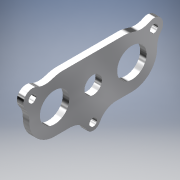
# Autodesk Inventor part: Gearbox Plate 1
Saved by Autodesk Inventor 2019.4 (Build 234330000, 330)
## iProperties
Created: 2019-12-11
Part Number: Gearbox Plate 1
Material: Aluminum 6061
Document SubType Name: Modeling
Designer: admin
Density: 2.7 g/cm^3
Appearance: Aluminum - Flat
Author: admin
Autodesk Inventor part; units mm, degrees
ref_plane "YZ Plane" through (0, 0, 0) normal (1, 0, 0) x (0, 1, 0)
ref_plane "XZ Plane" through (0, 0, 0) normal (0, 1, 0) x (-1, 0, 0)
ref_plane "XY Plane" through (0, 0, 0) normal (0, 0, 1) x (1, 0, 0)
sketch "Sketch6" plane through (0, 0, 0) normal (1, 0, 0) x (0, 1, 0)
  circle A0 centre (0, 0) radius 9.5
  circle A1 centre (0, -42) radius 16
  circle A2 centre (0, 42) radius 16
  line L0 (0, 0) -> (0, -14.5947) construction
  line L1 (0, 0) -> (0, -33.02)
  line L2 (0, 0) -> (33.02, 0) construction
  circle A3 centre (0, -33.02) radius 30
  line L3 (0, 0) -> (0, 33.02)
  line L4 (0, 0) -> (33.02, 0) construction
  circle A4 centre (0, 33.02) radius 30
  line L5 (0, 0) -> (0, -42)
  line L6 (0, 0) -> (0, 42)
  circle A5 centre (0, 42) radius 27.5
  circle A6 centre (0, -42) radius 27.5
  line L7 (30, 33.02) -> (30, -33.02)
  line L8 (-27.5, 42) -> (-27.5, -42)
  line L9 (26.4128, 49.6559) -> (28.814, 41.3719)
  line L10 (26.4128, -49.6559) -> (28.814, -41.3719)
  dimension "d45" = 19
  dimension "d46" = 32
  dimension "d47" = 32
  dimension "d50" = 0
  dimension "d51" = 0
  dimension "d52" = 33.02
  dimension "d53" = 90
  dimension "d54" = 60
  dimension "d55" = 33.02
  dimension "d56" = 90
  dimension "d57" = 60
  dimension "d58" = 42
  dimension "d59" = 42
  dimension "d60" = 55
  dimension "d61" = 55
  constraints: 22 end point, 8 point on circle, 7 centre point, 7 coincident, 7 tangent, 2 collinear, 2 horizontal, 2 perpendicular, 2 vertical
  measures "d45" diameter of A0
  measures "d46" diameter of A1
  measures "d47" diameter of A2
  measures "d50" distance from line of L0 A2.centre
  measures "d51" distance from line of A1.centre L0
  measures "d52" distance of L0.start L1.end
  measures "d53" angle of L1 L2
  measures "d54" diameter of A3
  measures "d55" distance of L0.start L3.end
  measures "d56" angle of L4 L3
  measures "d57" diameter of A4
  measures "d58" distance of L0.start L5.end
  measures "d59" distance of L0.start L6.end
  measures "d60" diameter of A5
  measures "d61" diameter of A6
extrude "Extrusion6" add sketch "Sketch6" along normal blind 7 contours A0 A3 L1 L3 A4 | A0 A4 L7 A3 | A4 L3 A0 | A0 L3 A5 A4 | A3 A6 L1 A0 | A0 L1 A3 | L3 A4 A0 | A0 A4 L8 A5 L3 | L3 L1 A3 A0 A4 | L1 A6 L8 A3 A0 | A0 A3 L1 | A0 A3 L8 A4 | A5 A4 | A4 A5 L9 | A6 A3 | L10 A6 A3 | A4 A5 | A6 A3 | A1 | A2
sketch "Sketch7" plane through (7, 0, 0) normal (1, 0, 0) x (0, 0, -1)
  circle A0 centre (0, 0) radius 9.5
  circle A1 centre (42, 0) radius 16
  circle A2 centre (-42, 0) radius 16
  line L0 (0, 0) -> (42, 0) construction
  line L1 (0, 0) -> (-42, 0) construction
  dimension "d64" = 19
  dimension "d65" = 32
  dimension "d66" = 32
  dimension "d67" = 0
  dimension "d69" = 0
  dimension "d70" = 42
  dimension "d71" = 42
  constraints: 5 end point, 3 centre point, 2 coincident
  measures "d64" diameter of A0
  measures "d65" diameter of A1
  measures "d66" diameter of A2
  measures "d67" vertical distance of L0.start A2.centre
  measures "d69" vertical distance of L0.end L0.start
  measures "d70" distance of L0.end L0.start
  measures "d71" distance of L0.start L1.end
extrude "Extrusion7" cut sketch "Sketch7" against normal blind 10
sketch "Sketch8" plane through (7, 0, 0) normal (1, 0, 0) x (0, 0, -1)
  circle A0 centre (-66.02, 20) radius 4.25 projected
  circle A1 centre (66.02, 20) radius 4.25 projected
  circle A2 centre (0, -35) radius 4 projected
  circle A3 centre (0, -35) radius 8
  circle A4 centre (-66.02, 20) radius 10
  circle A5 centre (66.02, 20) radius 10
  dimension "d82" = 16
  dimension "d83" = 20
  dimension "d84" = 20
  constraints: 3 centre point, 3 coincident
  measures "d82" diameter of A3
  measures "d83" diameter of A4
  measures "d84" diameter of A5
extrude "Extrusion8" add sketch "Sketch8" against normal blind 7
fillet "Fillet3" radius 20 6 edges at (3.5, 23.3137, 56.585) (3.5, 10.1208, 67.5699) (3.5, -27.5, -2.7839) (3.5, -27.5, 2.7839) (3.5, 23.3137, -56.585) (3.5, 10.1208, -67.5699)
sketch "Sketch9" plane through (7, 0, 0) normal (1, 0, 0) x (0, 0, -1)
  circle A0 centre (0, -35) radius 4.25 projected
  point P0 (0, 0)
extrude "Extrusion9" cut sketch "Sketch9" against normal blind 10
body "Solid2"
